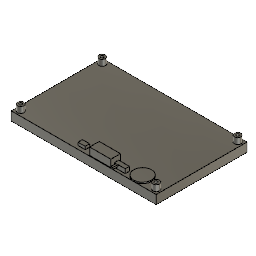
BTT_PITFT50_Mount_v6 (Autodesk Fusion 360 archive; units mm, degrees)
design "BTT PI TFT50 v2"
Autodesk Fusion 360 part; units mm, degrees
sketch "Sketch1" plane through (0, 0, 0) normal (0, 0, 1) x (1, 0, 0)
  line L0 (0, 0) -> (121, 0)
  line L1 (121, 0) -> (121, 76)
  line L2 (121, 76) -> (0, 76)
  line L3 (0, 76) -> (0, 0)
  circle A0 centre (4, 72) radius 2.75
  line L4 (0, 38) -> (121, 38) construction
  line L5 (60.5, 76) -> (60.5, 0) construction
  circle A1 centre (117, 72) radius 2.75
  circle A2 centre (4, 4) radius 2.75
  circle A3 centre (117, 4) radius 2.75
  circle A4 centre (103.2, 6.5) radius 7.5
  circle A5 centre (103.2, 6.5) radius 1
  line L6 (84, 5.7) -> (93, 5.7)
  line L7 (93, 5.7) -> (93, 2.2)
  line L8 (93, 2.2) -> (84, 2.2)
  line L9 (84, 2.2) -> (84, 5.7)
  line L10 (85.3592, 2.2) -> (86.8592, 2.2)
  line L11 (86.8592, 2.2) -> (86.8592, -2)
  line L12 (86.8592, -2) -> (85.3592, -2)
  line L13 (85.3592, -2) -> (85.3592, 2.2)
  line L14 (65, 8.5) -> (82.7, 8.5)
  line L15 (82.7, 8.5) -> (82.7, 0.5)
  line L16 (82.7, 0.5) -> (65, 0.5)
  line L17 (65, 0.5) -> (65, 8.5)
  line L18 (53, 2.8) -> (59, 2.8)
  line L19 (59, 2.8) -> (59, 6.5)
  line L20 (59, 6.5) -> (53, 6.5)
  line L21 (53, 6.5) -> (53, 2.8)
  circle A6 centre (4, 72) radius 1.25
  circle A7 centre (117, 72) radius 1.25
  circle A8 centre (4, 4) radius 1.25
  circle A9 centre (117, 4) radius 1.25
  dimension "d1" = 121
  dimension "d2" = 76
  dimension "d3" = 5.5
  dimension "d4" = 4
  dimension "d5" = 4
  dimension "d10" = 15
  dimension "d11" = 6.5
  dimension "d12" = 17.8
  dimension "d16" = 2
  dimension "d19" = 9
  dimension "d20" = 3.5
  dimension "d21" = 28
  dimension "d22" = 2.2
  dimension "d23" = 1.5
  dimension "d24" = 4.2
  dimension "d25" = 17.7
  dimension "d26" = 8
  dimension "d27" = 38.3
  dimension "d28" = 0.5
  dimension "d29" = 6
  dimension "d30" = 3.7
  dimension "d31" = 6
  dimension "d32" = 2.8
  dimension "d42" = -1.5
  dimension "d43" = 2.5
  constraint horizontal L0
  constraint vertical L1
  constraint horizontal L2
  constraint vertical L3
  constraint coincident L0.start L3.end
  constraint midpoint L3 L4.start
  constraint midpoint L1 L4.end
  constraint midpoint L2 L5.start
  constraint midpoint L0 L5.end
  constraint symmetric A0 L5 A1
  constraint symmetric A0 L4 A2
  constraint symmetric L4 A1 A3
  constraint concentric A4 A5
  constraint horizontal L6
  constraint vertical L7
  constraint horizontal L8
  constraint vertical L9
  constraint horizontal L10
  constraint vertical L11
  constraint horizontal L12
  constraint vertical L13
  constraint coincident L8 L10.start
  constraint horizontal L14
  constraint vertical L15
  constraint horizontal L16
  constraint vertical L17
  constraint horizontal L18
  constraint vertical L19
  constraint horizontal L20
  constraint vertical L21
  constraint symmetric L5 A6 A7
  constraint concentric A2 A8
  constraint symmetric L5 A8 A9
  measures "d1" distance of L0.start L0.end
  measures "d2" distance of L0.start L2.end
  measures "d3" diameter of A0
  measures "d4" distance of L2 A0.centre
  measures "d5" distance of L3 A0.centre
  measures "d10" diameter of A4
  measures "d11" distance of L0 A4.centre
  measures "d12" distance of L1 A4.centre
  measures "d16" diameter of A5
  measures "d19" distance of L6.start L6.end
  measures "d20" distance of L6.start L8.end
  measures "d21" distance of L1 L7
  measures "d22" distance of L0 L8
  measures "d23" distance of L10.start L10.end
  measures "d24" distance of L10.start L12.end
  measures "d25" distance of L14.start L14.end
  measures "d26" distance of L14.start L16.end
  measures "d27" distance of L1 L15
  measures "d28" distance of L0 L16
  measures "d29" distance of L18.start L18.end
  measures "d30" distance of L18.start L20.end
  measures "d31" distance of L17 L19
  measures "d32" distance of L0 L18
  measures "d43" diameter of A8
extrude "Extrude1" add sketch "Sketch1" against normal blind 7.5 contours L0 L1 L2 L3 A4 L6 L7 L8 L9 L11 L13 | L0 L8 L10 L11 L13 | L6 L7 L8 L9 L10 | L0 A4 | A0 | A1 | A2 | A3 | A5 | L14 L15 L16 L17 | L18 L19 L20 L21 | A6 | A7 | A8 | A9 picked at (103.2249, 1.8343) makes body 1
extrude "Extrude2" add sketch "Sketch1" along normal blind 5 contours A0 | A1 | A2 | A3 | A6 | A7 | A8 | A9 bodies 1
extrude "Extrude3" add sketch "Sketch1" along normal blind 1 from surface at 1 separate body contours L0 A4 | L0 A4 | A5 makes body 2
extrude "Extrude4" add sketch "Sketch1" along normal blind 2 contours A5 bodies 2 1
extrude "Extrude5" add sketch "Sketch1" along normal blind 3.5 contours L6 L7 L8 L9 L10 bodies 2
extrude "Extrude6" add sketch "Sketch1" along normal blind 1.5 from surface at 2 contours L0 L8 L10 L11 L13 | L0 L11 L12 L13 bodies 2
extrude "Extrude7" add sketch "Sketch1" along normal blind 6.1 contours L14 L15 L16 L17 bodies 2
extrude "Extrude8" add sketch "Sketch1" along normal blind 2.4 contours L18 L19 L20 L21 bodies 2
extrude "Extrude9" cut sketch "Sketch1" along normal blind 4 from surface at 1 contours A6 | A7 | A8 | A9 bodies 2
